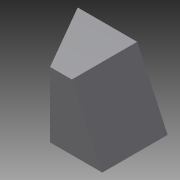
# Autodesk Inventor part: lesson2
Saved by Autodesk Inventor 2011 SP1 (Build 150282100, 282)
## iProperties
Created: 2011-10-07
Part Number: lesson2
Document SubType Name: Modeling
Designer: Kevin
Density: 1 g/cm^3
Author: Kevin
Autodesk Inventor part; units mm, degrees
ref_plane "YZ Plane" through (0, 0, 0) normal (1, 0, 0) x (0, 1, 0)
ref_plane "XZ Plane" through (0, 0, 0) normal (0, 1, 0) x (-1, 0, 0)
ref_plane "XY Plane" through (0, 0, 0) normal (0, 0, 1) x (1, 0, 0)
sketch "Sketch1" plane through (0, 0, 0) normal (0, 0, 1) x (1, 0, 0)
  line L0 (-12.7022, 10.8383) -> (10.9581, 10.8383)
  line L1 (10.9581, 10.8383) -> (10.9581, -4.1617)
  line L2 (10.9581, -4.1617) -> (-4.0419, -4.1617)
  line L3 (-4.0419, -4.1617) -> (-12.7022, 10.8383)
  point P0 (0, 0)
  dimension "d0" = 15
  dimension "d1" = 15
  dimension "d3" = 120
  constraints: 8 end point, 1 horizontal, 1 parallel, 1 perpendicular
  measures "d0" distance of L0.end L1.end
  measures "d1" distance of L1.end L2.end
  measures "d3" angle of L2 L3
extrude "Extrusion1" add sketch "Sketch1" along normal blind 15
sketch "Sketch2" plane through (-4.0419, -4.1617, 0) normal (0, -1, 0) x (1, 0, 0)
  line L0 (15, 15) -> (0, 15) projected
  line L1 (15, 0) -> (0, 0) projected
  line L2 (15, 0) -> (15, 15) projected
  line L3 (5, 15) -> (11.9946, 0)
  point P0 (4.0419, 0)
  dimension "d6" = 5
  dimension "d7" = 65
  constraints: 2 end point, 2 point on line
  measures "d6" distance of L3.start L0.end
  measures "d7" angle of L3 L1
extrude "Extrusion2" cut sketch "Sketch2" against normal through all
body "Solid1"
